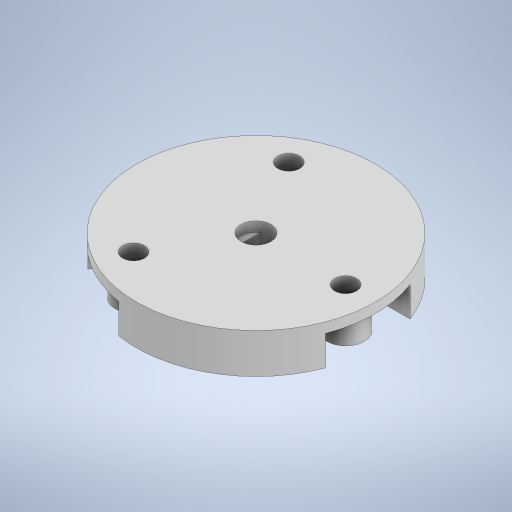
# Autodesk Inventor part: Soporte rodamientos
Saved by Autodesk Inventor 2023 (Build 270158000, 158)
## iProperties
Created: 2023-04-01
Part Number: Soporte rodamientos
Material: Genérico
Document SubType Name: Modeling
Designer: sergi
Density: 1 g/cm^3
Appearance: Valor por defecto
Author: sergi
Autodesk Inventor part; units mm, degrees
ref_plane "YZ Plane" through (0, 0, 0) normal (1, 0, 0) x (0, 1, 0)
ref_plane "XZ Plane" through (0, 0, 0) normal (0, 1, 0) x (-1, 0, 0)
ref_plane "XY Plane" through (0, 0, 0) normal (0, 0, 1) x (1, 0, 0)
sketch "Boceto1" plane through (0, 0, 0) normal (0, 1, 0) x (-1, 0, 0)
  circle A0 centre (0, 0) radius 24
  dimension "d0" = 48
  constraints: 1 centre point, 1 coincident
  measures "d0" diameter of A0
extrude "Extrusión1" add sketch "Boceto1" along normal blind 8
sketch "Boceto2" plane through (0, 8, 0) normal (0, 1, 0) x (1, 0, 0)
  circle A0 centre (0, 0) radius 3
  line L0 (0, 0) -> (-1.6, 0)
  line L1 (-1.6, 0) -> (-1.6, -2.5377)
  line L2 (-1.6, 2.5377) -> (-1.6, 0)
  line L3 (1.6, 2.5377) -> (1.6, -2.5377)
  dimension "d3" = 6
  dimension "d4" = 1.6
  constraints: 8 end point, 4 point on circle, 1 centre point, 1 coincident, 1 collinear, 1 horizontal, 1 parallel, 1 perpendicular, 1 point on line
  measures "d3" diameter of A0
  measures "d4" distance of L0.start L0.end
extrude "Extrusión2" cut sketch "Boceto2" against normal through all contours L3 A0 L1 L2
sketch "Boceto3" plane through (0, 8, 0) normal (0, 1, 0) x (1, 0, 0)
  circle A0 centre (0, 0) radius 3
  constraints: 1 centre point, 1 coincident
extrude "Extrusión3" cut sketch "Boceto3" against normal blind 2
sketch "Boceto5" plane through (0, 0, 0) normal (0, -1, 0) x (1, 0, 0)
  line L0 (0, 0) -> (26, 0)
  line L1 (26, 0) -> (18, 0)
  circle A0 centre (18, 0) radius 8.5
  circle A1 centre (18, 0) radius 3.75
  line L2 (18, -8.5) -> (26.5, -8.5)
  line L3 (26.5, -8.5) -> (26.5, 8.5)
  line L4 (26.5, 8.5) -> (18, 8.5)
  point P0 (26.5, 0)
  dimension "d12" = 26
  dimension "d13" = 8
  dimension "d14" = 17
  dimension "d15" = 7.5
  constraints: 10 end point, 2 centre point, 2 coincident, 2 horizontal, 2 perpendicular, 2 point on circle, 1 point on line, 1 tangent
  measures "d12" distance of L0.start L0.end
  measures "d13" distance of L0.end L1.end
  measures "d14" diameter of A0
  measures "d15" diameter of A1
extrude "Extrusión4" cut sketch "Boceto5" against normal blind 6
pattern_circular "Patrón circular1" count 3 over 360 about axis through (0, 0, 0) along (0, 1, 0) of "Extrusión4"
sketch "Boceto7" plane through (-9, 0, -15.5885) normal (0, -1, 0) x (1, 0, 0)
  circle A0 centre (0, 0) radius 3.75 projected
  circle A1 centre (0, 31.1769) radius 3.75 projected
  circle A2 centre (27, 15.5885) radius 3.75 projected
  point P0 (9, 15.5885)
  constraints: 3 coincident
hole "Agujero1" at (-9, 0, -15.5885) at (-9, 0, 15.5885) at (18, 0, 0) direction (0, 1, 0) diameter 4.4 end through all
